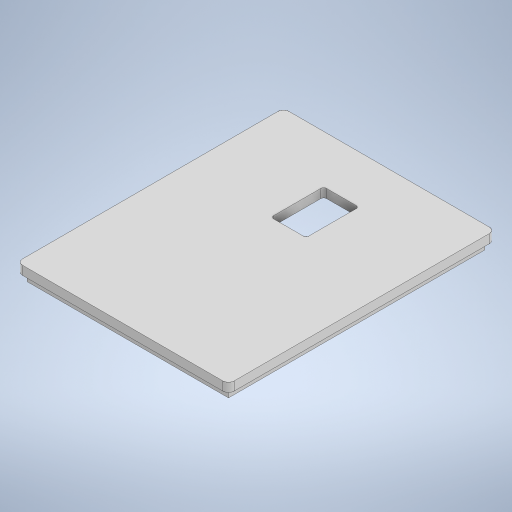
# Autodesk Inventor part: Light Sensor Cover V1
Saved by Autodesk Inventor 2024.2 (Build 282272000, 272)
## iProperties
Created: 2024-07-12
Part Number: Light Sensor Cover V1
Material: Generic
Document SubType Name: Modeling
Designer: balmo
Density: 1 g/cm^3
Appearance: Default
Author: balmo
## iProperties of the stored document Light Sensor Cover V1_3DPrint.ipt
Created: 2024-07-12
Part Number: Light Sensor Cover V1_3DPrint
Material: Generic
Document SubType Name: Modeling
Designer: balmo
Density: 1 g/cm^3
Appearance: Default
Author: balmo
Autodesk Inventor part; units mm, degrees
ref_plane "YZ Plane" through (0, 0, 0) normal (1, 0, 0) x (0, 1, 0)
ref_plane "XZ Plane" through (0, 0, 0) normal (0, 1, 0) x (-1, 0, 0)
ref_plane "XY Plane" through (0, 0, 0) normal (0, 0, 1) x (1, 0, 0)
sketch "Sketch1" plane through (0, 0, 0) normal (0, 1, 0) x (-1, 0, 0)
  line L0 (0, 0) -> (19.05, 0)
  line L1 (19.05, 0) -> (19.05, -24.003)
  line L2 (19.05, -24.003) -> (0, -24.003)
  line L3 (0, -24.003) -> (0, 0)
  dimension "d0" = 24.003
  dimension "d1" = 19.05
  constraints: 8 end point, 2 parallel, 1 horizontal, 1 perpendicular
  measures "d0" distance between parallel lines of L2 L0
  measures "d1" distance between parallel lines of L3 L1
extrude "Extrusion1" add sketch "Sketch1" against normal blind 0.7937
fillet "Fillet1" radius 0.508 4 edges at (0, -0.3969, 0) (-19.05, -0.3969, 0) (0, -0.3969, -24.003) (-19.05, -0.3969, -24.003)
sketch "Sketch2" plane through (0, -0.7937, 0) normal (0, -1, 0) x (1, 0, 0)
  line L0 (-18.542, -24.003) -> (-0.508, -24.003) projected
  line L1 (0, -23.495) -> (0, -0.508) projected
  line L2 (-0.508, 0) -> (-18.542, 0) projected
  line L3 (-19.05, -0.508) -> (-19.05, -23.495) projected
  line L4 (-0.4572, -0.4572) -> (-18.5928, -0.4572)
  line L5 (-18.5928, -0.4572) -> (-18.5928, -23.5458)
  line L6 (-18.5928, -23.5458) -> (-0.4572, -23.5458)
  line L7 (-0.4572, -23.5458) -> (-0.4572, -0.4572)
  line L8 (-1.143, -1.143) -> (-17.907, -1.143)
  line L9 (-17.907, -1.143) -> (-17.907, -22.86)
  line L10 (-17.907, -22.86) -> (-1.143, -22.86)
  line L11 (-1.143, -22.86) -> (-1.143, -1.143)
  arc A0 (-19.05, -23.495) -> (-18.542, -24.003) centre (-18.542, -23.495) ccw projected
  arc A1 (-0.508, -24.003) -> (0, -23.495) centre (-0.508, -23.495) ccw projected
  arc A2 (0, -0.508) -> (-0.508, 0) centre (-0.508, -0.508) ccw projected
  arc A3 (-18.542, 0) -> (-19.05, -0.508) centre (-18.542, -0.508) ccw projected
  point P0 (0, 0)
  dimension "d5" = 0.4572
  dimension "d6" = 0.4572
  dimension "d7" = 0.4572
  dimension "d8" = 0.4572
  dimension "d9" = 1.143
  dimension "d10" = 1.143
  dimension "d11" = 1.143
  dimension "d12" = 1.143
  constraints: 16 end point, 4 parallel, 2 horizontal, 2 perpendicular
  measures "d5" distance between parallel lines of L5 L3
  measures "d6" distance between parallel lines of L2 L4
  measures "d7" distance between parallel lines of L1 L7
  measures "d8" distance between parallel lines of L6 L0
  measures "d9" distance between parallel lines of L11 L1
  measures "d10" distance between parallel lines of L8 L2
  measures "d11" distance between parallel lines of L9 L3
  measures "d12" distance between parallel lines of L10 L0
extrude "Extrusion2" add sketch "Sketch2" along normal blind 0.7366 contours L7 L6 L5 L4
sketch "Sketch3" plane through (0, 0, 0) normal (0, 1, 0) x (1, 0, 0)
  arc A0 (-18.542, 24.003) -> (-19.05, 23.495) centre (-18.542, 23.495) ccw projected
  line L0 (-19.05, 23.495) -> (-19.05, 0.508) projected
  arc A1 (-19.05, 0.508) -> (-18.542, 0) centre (-18.542, 0.508) ccw projected
  line L1 (-18.542, 0) -> (-0.508, 0) projected
  arc A2 (-0.508, 0) -> (0, 0.508) centre (-0.508, 0.508) ccw projected
  line L2 (0, 0.508) -> (0, 23.495) projected
  arc A3 (0, 23.495) -> (-0.508, 24.003) centre (-0.508, 23.495) ccw projected
  line L3 (-0.508, 24.003) -> (-18.542, 24.003) projected
  line L4 (-11.1125, 19.685) -> (-7.9375, 19.685)
  line L5 (-7.9375, 19.685) -> (-7.9375, 14.9225)
  line L6 (-7.9375, 14.9225) -> (-11.1125, 14.9225)
  line L7 (-11.1125, 14.9225) -> (-11.1125, 19.685)
  point P0 (0, 0)
  dimension "d15" = 3.175
  dimension "d16" = 4.7625
  dimension "d17" = 19.05
  dimension "d18" = 7.9375
  dimension "d19" = 7.9375
  dimension "d20" = 4.318
  constraints: 8 end point, 2 parallel, 1 horizontal, 1 perpendicular
  measures "d15" distance of L5.end L6.end
  measures "d16" distance of L4.end L5.end
  measures "d17" distance between parallel lines of L2 L0
  measures "d18" distance between parallel lines of L0 L7
  measures "d19" distance between parallel lines of L5 L2
  measures "d20" distance between parallel lines of L3 L4
extrude "Extrusion3" cut sketch "Sketch3" against normal blind 3.9116 contours L4 L5 L6 L7
fillet "Fillet2" radius 0.254 4 edges at (-11.1125, -0.3969, -19.685) (-7.9375, -0.3969, -19.685) (-7.9375, -0.3969, -14.9225) (-11.1125, -0.3969, -14.9225)
body "Solid1"
